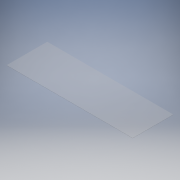
# Autodesk Inventor part: Bottom
Saved by Autodesk Inventor 2017 (Build 210142000, 142)
## iProperties
Created: 2017-01-16
Part Number: Bottom
Material: Polycarbonate, Clear
Document SubType Name: Modeling
Designer: Ben
Density: 1.2 g/cm^3
Appearance: Polycarbonate - Clear
Mass: 350.504 g
Surface Area: 3711.28 cm^2
Volume: 292.087 cm^3
Author: Ben
Autodesk Inventor part; units mm, degrees
ref_plane "YZ Plane" through (0, 0, 0) normal (1, 0, 0) x (0, 1, 0)
ref_plane "XZ Plane" through (0, 0, 0) normal (0, 1, 0) x (-1, 0, 0)
ref_plane "XY Plane" through (0, 0, 0) normal (0, 0, 1) x (1, 0, 0)
sketch "Sketch1" plane through (0, 0, 0) normal (0, 1, 0) x (-1, 0, 0)
  line L0 (-384.175, 0) -> (-384.175, -247.65)
  line L1 (-384.175, -247.65) -> (384.175, -247.65)
  line L2 (384.175, -247.65) -> (384.175, 0)
  line L3 (384.175, 0) -> (-384.175, 0)
  point P0 (0, 0)
  point P1 (0, 0)
  dimension "d0" = 247.65
  dimension "d2" = 768.35
  constraints: 8 end point, 2 horizontal, 1 coincident, 1 midpoint, 1 parallel, 1 vertical
  measures "d0" distance of L2.end L1.end
  measures "d2" distance of L2.end L0.start
extrude "Extrusion1" add sketch "Sketch1" along normal blind 1.5875
body "Solid1"
